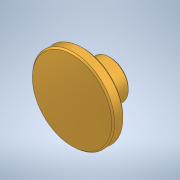
# Autodesk Inventor part: EW_Drehknopf
Saved by Autodesk Inventor 2020 (Build 240168000, 168)
## iProperties
Created: 2020-06-21
Part Number: EW_Drehknopf
Material: Messing, weicher Gelbton
Document SubType Name: Modeling
Designer: Johannes
Density: 8.47 g/cm^3
Appearance: Messing - satiniert
Author: Johannes
Autodesk Inventor part; units mm, degrees
ref_plane "YZ Plane" through (0, 0, 0) normal (1, 0, 0) x (0, 1, 0)
ref_plane "XZ Plane" through (0, 0, 0) normal (0, 1, 0) x (-1, 0, 0)
ref_plane "XY Plane" through (0, 0, 0) normal (0, 0, 1) x (1, 0, 0)
sketch "Skizze1" plane through (0, 0, 0) normal (1, 0, 0) x (0, 1, 0)
  line L0 (0, 0) -> (0, 67.4576) construction
  line L1 (3, 0) -> (3, 12)
  line L2 (3, 12) -> (0, 12)
  line L3 (0, 12) -> (0, 15)
  line L4 (15, 14) -> (15, 10)
  line L5 (7, 6) -> (7, 0)
  line L6 (7, 0) -> (3, 0)
  arc A0 (15, 10) -> (7, 6) centre (15, 0) ccw
  line L7 (15, 10) -> (23.1737, 10) construction
  arc A1 (15, 14) -> (0, 15) centre (0, -98) ccw
  line L8 (0, 15) -> (-13.142, 15) construction
  dimension "d0" = 6
  dimension "d1" = 14
  dimension "d2" = 30
  dimension "d3" = 6
  dimension "d5" = 4
  dimension "d6" = 12
  dimension "d12" = 10
  dimension "d13" = 15
  constraints: 18 end point, 5 vertical, 4 horizontal, 4 point on circle, 2 centre point, 2 point on line, 2 tangent
  measures "d0" diameter of L1 L0
  measures "d1" diameter of L5 L0
  measures "d2" diameter of L4 L0
  measures "d3" distance of L5.start L5.end
  measures "d5" distance of L4.start L4.end
  measures "d6" distance of L1.start L1.end
  measures "d12" vertical distance of L4.end L5.end
  measures "d13" distance from line of L0.start L8
revolve "Umdrehung1" add sketch "Skizze1" angle 360 about axis through (0, 0, 0) along (0, 0, 1)
chamfer "Fase1" distance 0.5 angle 45 4 edges at (0, -7, 0) (0, -3, 0) (0, -15, 10) (0, -15, 14)
sketch "Skizze2" plane through (0, 0, 0) normal (0, 1, 0) x (-1, 0, 0)
  line L0 (6.5, 0) -> (-6.5, 0) projected
  point P0 (0, 0)
  point P1 (0, 2.5)
  point P2 (0, 0)
  dimension "d14" = 2.5
  constraints: 1 midpoint, 1 vertical alignment
  measures "d14" distance from line of L0 point (0, 2.5)
hole "Bohrung1" at (0, 0, 2.5) direction (0, -1, 0) diameter 2.459 end through all thread size "M3x0.5" class "6H" standard "ISO Metric profile"
